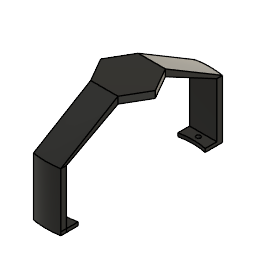
cover_plate (Autodesk Fusion 360 design; units mm, degrees)
part number: 2026-05-21-21-22-30-375
Autodesk Fusion 360 part; units mm, degrees
sketch "Sketch1" plane through (0, 0, 0) normal (0, 0, 1) x (1, 0, 0)
  circle A0 centre (0, 0) radius 60
  dimension "d1" = 120
  constraint coincident A0.centre origin
  measures "d1" diameter of A0
extrude "Extrude1" add sketch "Sketch1" along normal blind 2.5 makes body 1
sketch "Sketch2" plane through (0, 0, 2.5) normal (0, 0, 1) x (-1, 0, 0)
  circle A0 centre (0, 0) radius 60
  line L0 (0, 0) -> (0, -60)
  line L1 (0, 0) -> (0, 60)
  circle A1 centre (0, 0) radius 45
  line L2 (0, -45) -> (-10, -45)
  line L3 (0, -45) -> (10, -45)
  line L4 (10, -45) -> (10, -59.1608)
  line L5 (-10, -45) -> (-10, -59.1608)
  line L6 (0, 45) -> (-10, 45)
  line L7 (0, 45) -> (10, 45)
  line L8 (10, 45) -> (10, 59.1608)
  line L9 (-10, 45) -> (-10, 59.1608)
  line L10 (0, -60) -> (0, -55)
  line L11 (0, -55) -> (-10, -55)
  line L12 (0, -55) -> (10, -55)
  line L13 (0, 60) -> (0, 55)
  line L14 (-10, 55) -> (0, 55)
  line L15 (0, 55) -> (10, 55)
  dimension "d5" = 90
  dimension "d6" = 10
  dimension "d7" = 10
  dimension "d8" = 10
  dimension "d9" = 10
  constraint coincident A0 L0.end
  constraint vertical L0
  constraint coincident A0 L1.end
  constraint parallel L0 L1
  constraint concentric A0 A1
  constraint coincident A1 L2.start
  constraint coincident L0 L2.start
  constraint perpendicular L0 L2
  constraint perpendicular L0 L3
  constraint coincident A0 L4.end
  constraint perpendicular L3 L4
  constraint coincident A0 L5.end
  constraint perpendicular L2 L5
  constraint coincident A1 L6.start
  constraint perpendicular L1 L6
  constraint perpendicular L1 L7
  constraint coincident A0 L8.end
  constraint perpendicular L7 L8
  constraint coincident A0 L9.end
  constraint perpendicular L6 L9
  constraint coincident L0 L10.end
  constraint coincident L5 L11.end
  constraint perpendicular L5 L11
  constraint coincident L4 L12.end
  constraint perpendicular L4 L12
  constraint coincident L1 L13.end
  constraint coincident L9 L14.start
  constraint perpendicular L1 L14
  constraint coincident L8 L15.end
  constraint perpendicular L8 L15
  measures "d5" diameter of A1
  measures "d6" distance of L2.start L2.end
  measures "d7" distance of L2.start L3.end
  measures "d8" distance of L6.start L6.end
  measures "d9" distance of L6.start L7.end
extrude "Extrude2" add sketch "Sketch2" along normal blind 40 contours A0 L1 L8 L13 L15 | A0 L0 L4 L10 L12 | A0 L1 L9 L13 L14 | A0 L0 L5 L10 L11 bodies 1
sketch "Sketch3" plane through (0, 0, 0) normal (1, 0, 0) x (0, 1, 0)
  line L0 (-0.0059, 2.4931) -> (-0.0059, 62.4931)
  line L1 (-0.0059, 62.4931) -> (24.9941, 62.4931)
  line L2 (24.9941, 62.4931) -> (-0.0059, 62.4931)
  line L3 (-0.0059, 62.4931) -> (-25.0059, 62.4931)
  line L4 (-25.0059, 62.4931) -> (-25.0059, 67.4931)
  line L5 (-25.0059, 67.4931) -> (24.9941, 67.4931)
  line L6 (24.9941, 67.4931) -> (24.9941, 62.4931)
  dimension "d12" = 60
  dimension "d13" = 25
  dimension "d14" = 25
  dimension "d15" = 5
  dimension "d16" = 50
  constraint vertical L0
  constraint perpendicular L0 L1
  constraint perpendicular L0 L3
  constraint perpendicular L3 L4
  constraint perpendicular L4 L5
  measures "d12" distance of L0.start L0.end
  measures "d13" distance of L0.end L1.end
  measures "d14" distance of L0.end L3.end
  measures "d15" distance of L3.end L4.end
  measures "d16" distance of L4.end L5.end
extrude "Extrude3" add sketch "Sketch3" along normal blind 20 separate body makes body 2
extrude "Extrude4" add 1 faces at (0, -0.0059, 65.8264) along direction (-1, 0, 0) blind 20 on bodies 2 bodies 2
sketch "Sketch4" plane through (0, 0, 67.4931) normal (0, 0, 1) x (-1, 0, 0)
  line L0 (20, 25.0059) -> (-20, 25.0059)
  line L1 (-20, 25.0059) -> (-20, -24.9941)
  line L2 (-20, -24.9941) -> (20, -24.9941)
  line L3 (20, -24.9941) -> (20, 25.0059)
  line L4 (-9.9944, 17.3237) -> (-20, 0.0064)
  line L5 (-20, 0.0064) -> (-10.0055, -17.3173)
  line L6 (-10.0055, -17.3173) -> (9.9944, -17.3237)
  line L7 (9.9944, -17.3237) -> (20, -0.0064)
  line L8 (20, -0.0064) -> (10.0055, 17.3173)
  line L9 (10.0055, 17.3173) -> (-9.9944, 17.3237)
  dimension "d21" = 20
  measures "d21" distance of L4.start origin
extrude "Extrude5" cut sketch "Sketch4" against normal blind 10 contours L0 L1 L3 L4 L8 L9 | L1 L2 L3 L5 L6 L7 bodies 2
loft "Loft1" add section 1 face at (1.1157, 56.6355, 42.5) section 2 face at (3.3389, 17.3194, 65.8264) on bodies 1 2 bodies 1 2
loft "Loft2" add section 1 face at (-3.3389, -17.3194, 64.1597) section 2 face at (1.1157, -56.6355, 42.5) on bodies 1 bodies 1
sketch "Sketch5" plane through (0, 0, 2.5) normal (0, 0, 1) x (-1, 0, 0)
  line L0 (10, -55) -> (10, -59.1608)
  arc A0 (10, -59.1608) -> (10, 59.1608) centre (0, 0) ccw
  line L1 (10, 59.1608) -> (10, 55)
  line L2 (10, 55) -> (-10, 55)
  line L3 (-10, 55) -> (-10, 59.1608)
  arc A1 (-10, 59.1608) -> (-10, -59.1608) centre (0, 0) ccw
  line L4 (-10, -59.1608) -> (-10, -55)
  line L5 (-10, -55) -> (10, -55)
  circle A2 centre (0, 0) radius 47.5
  line L6 (0, -47.5) -> (0, -51.5)
  line L7 (10, -55) -> (10, -46.4354)
  line L8 (-10, -55) -> (-10, -46.4354)
  line L9 (10, -55) -> (10, -59.1608)
  line L10 (-10, -55) -> (-10, -59.1608)
  line L11 (-10, 55) -> (-10, 46.4354)
  line L12 (10, 55) -> (10, 46.4354)
  line L13 (0, 47.5) -> (0, 51.5)
  circle A3 centre (0, -51.5) radius 1.6
  circle A4 centre (0, 51.5) radius 1.6
  dimension "d24" = 95
  dimension "d27" = 3.2
  dimension "d28" = 3.2
  constraint concentric A0 A2
  constraint coincident A2 L6.start
  constraint perpendicular L5 L6
  constraint coincident L0.start L5.end
  constraint coincident A2 L7.end
  constraint perpendicular L5 L7
  constraint coincident L4.end L5.start
  constraint coincident A2 L8.end
  constraint perpendicular L5 L8
  constraint coincident L0.end A0.start
  constraint coincident A1.end L4.start
  constraint coincident L2.end L3.start
  constraint coincident A2 L11.end
  constraint perpendicular L2 L11
  constraint coincident L1.end L2.start
  constraint coincident A2 L12.end
  constraint perpendicular L2 L12
  constraint coincident A2 L13.start
  constraint perpendicular L2 L13
  constraint coincident L6.end A3.centre
  constraint coincident L13.end A4.centre
  measures "d24" diameter of A2
  measures "d27" diameter of A3
  measures "d28" diameter of A4
extrude "Extrude6" cut sketch "Sketch5" against normal blind 10 contours L0 A0 L1 A2 L7 L9 L12 | L3 A1 L4 A2 L8 L10 L11 | A2 | A3 | A4 bodies 1
